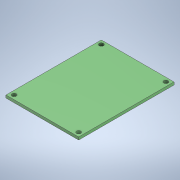
# Autodesk Inventor part: Mock Module PCB
Saved by Autodesk Inventor 2022 (Build 260153000, 153)
## iProperties
Created: 2021-07-19
Part Number: Mock Module PCB
Material: Generic
Document SubType Name: Modeling
Designer: Caleb
Density: 1 g/cm^3
Appearance: Default
Author: Caleb
Autodesk Inventor part; units mm, degrees
ref_plane "YZ Plane" through (0, 0, 0) normal (1, 0, 0) x (0, 1, 0)
ref_plane "XZ Plane" through (0, 0, 0) normal (0, 1, 0) x (-1, 0, 0)
ref_plane "XY Plane" through (0, 0, 0) normal (0, 0, 1) x (1, 0, 0)
sketch "Sketch1" plane through (0, 0, 0) normal (0, 1, 0) x (-1, 0, 0)
  line L0 (-21.5, 28.2) -> (21.5, 28.2)
  line L1 (21.5, 28.2) -> (21.5, -28.2)
  line L2 (21.5, -28.2) -> (-21.5, -28.2)
  line L3 (-21.5, -28.2) -> (-21.5, 28.2)
  line L4 (-21.5, 28.2) -> (21.5, -28.2) construction
  line L5 (21.5, 28.2) -> (-21.5, -28.2) construction
  point P0 (0, 0)
  dimension "d0" = 43
  dimension "d1" = 56.4
  constraints: 12 end point, 2 midpoint, 2 parallel, 1 horizontal, 1 perpendicular
  measures "d0" distance of L0.start L0.end
  measures "d1" distance of L0.end L1.end
extrude "Extrusion1" add sketch "Sketch1" along normal blind 1.6
sketch "Sketch2" plane through (0, 1.6, 0) normal (0, 1, 0) x (1, 0, 0)
  point P0 (0, 0)
  point P1 (-19.1, -25.8)
  point P2 (-19.1, 25.8)
  point P3 (19.1, 25.8)
  point P4 (19.1, -25.8)
  dimension "d4" = 25.8
  dimension "d5" = 19.1
  dimension "d6" = 19.1
  dimension "d7" = 25.8
  constraints: 2 horizontal alignment, 2 vertical alignment
  measures "d4" vertical distance of point (-19.1, -25.8) point (0, 0)
  measures "d5" horizontal distance of point (-19.1, -25.8) point (0, 0)
  measures "d6" horizontal distance of point (19.1, 25.8) point (0, 0)
  measures "d7" vertical distance of point (19.1, 25.8) point (0, 0)
hole "Hole1" at (-19.1, 1.6, 25.8) at (-19.1, 1.6, -25.8) at (19.1, 1.6, -25.8) at (19.1, 1.6, 25.8) direction (0, -1, 0) diameter 2.5 end through all
body "Solid1"
